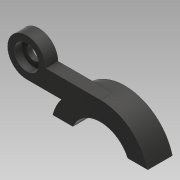
# Autodesk Inventor part: CameraMount
Saved by Autodesk Inventor 2020.3 (Build 243373000, 373)
## iProperties
Created: 2021-10-17
Part Number: CameraMount
Material: ABS Plastic
Document SubType Name: Modeling
Designer: justi
Density: 1.06 g/cm^3
Appearance: Smooth - Black
Author: justi
Autodesk Inventor part; units mm, degrees
ref_plane "YZ Plane" through (0, 0, 0) normal (1, 0, 0) x (0, 1, 0)
ref_plane "XZ Plane" through (0, 0, 0) normal (0, 1, 0) x (-1, 0, 0)
ref_plane "XY Plane" through (0, 0, 0) normal (0, 0, 1) x (1, 0, 0)
sketch "Sketch1" plane through (0, 0, 0) normal (0, 1, 0) x (-1, 0, 0)
  circle A0 centre (0, 0) radius 2.75
  arc A1 (0, -7.75) -> (-7.75, 0) centre (0, 0) ccw
  line L0 (0, 0) -> (-30, 0)
  line L1 (0, -7.75) -> (-14.1906, -7.75)
  line L2 (-30, 0) -> (-30, -20) construction
  arc A2 (-18.8169, -15) -> (-41.1831, -15) centre (-30, -20) ccw
  line L3 (-30, 0) -> (-30, -15) construction
  line L4 (-41.1831, -15) -> (-49.3649, -15)
  line L5 (-18.8169, -15) -> (-10.6351, -15)
  arc A3 (-10.6351, -15) -> (-14.1906, -7.75) centre (-30, -20) ccw
  arc A4 (-30, 0) -> (-49.3649, -15) centre (-30, -20) ccw
  dimension "d0" = 5.5
  dimension "d1" = 5
  dimension "d2" = 30
  dimension "d3" = 20
  dimension "d4" = 15
  constraints: 12 end point, 8 point on circle, 5 centre point, 3 coincident, 3 perpendicular, 2 horizontal, 2 point on line, 1 tangent
  measures "d0" diameter of A0
  measures "d1" radial gap between concentric circles of A0 A1
  measures "d2" distance of L0.start L0.end
  measures "d3" distance of L0.end L2.end
  measures "d4" distance of L0.end L3.end
extrude "Extrusion1" add sketch "Sketch1" along normal blind 5
sketch "Sketch2" plane through (0, 5, 0) normal (0, 1, 0) x (1, 0, 0)
  arc A0 (18.8169, 15) -> (41.1831, 15) centre (30, 20) ccw projected
  circle A1 centre (30, 20) radius 12.25
  line L0 (7.75, 0) -> (30, 0) projected
  circle A2 centre (30, 20) radius 20
  line L1 (49.3649, 15) -> (41.1831, 15) projected
  line L2 (49.3649, 15) -> (10.6351, 15)
  point P0 (0, 0)
  constraints: 3 coincident, 2 centre point, 2 end point, 2 point on circle, 1 collinear, 1 concentric
extrude "Extrusion2" add sketch "Sketch2" along normal blind 5 contours A0 L1 A2 L2
sketch "Sketch3" plane through (0, 0, 0) normal (0, -1, 0) x (1, 0, 0)
  circle A0 centre (0, 0) radius 5
  dimension "d9" = 10
  constraints: 1 centre point, 1 coincident
  measures "d9" diameter of A0
extrude "Extrusion3" cut sketch "Sketch3" against normal blind 3
body "Solid1"
